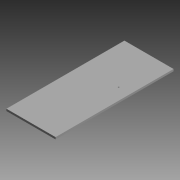
# Autodesk Inventor part: Wand rechts_CPY
Saved by Autodesk Inventor 2013 (Build 170138000, 138)
## iProperties
Created: 2012-10-20
Part Number: Wand rechts_CPY
Material: Allgemein
Document SubType Name: Modeling
Designer: fivef
Density: 1 g/cm^3
Author: fivef
Autodesk Inventor part; units mm, degrees
ref_plane "YZ Plane" through (0, 0, 0) normal (1, 0, 0) x (0, 1, 0)
ref_plane "XZ Plane" through (0, 0, 0) normal (0, 1, 0) x (-1, 0, 0)
ref_plane "XY Plane" through (0, 0, 0) normal (0, 0, 1) x (1, 0, 0)
sketch "Skizze1" plane through (0, 0, 0) normal (0, 0, 1) x (1, 0, 0)
  line L0 (0, 215.5102) -> (250, 215.5102)
  line L1 (250, 215.5102) -> (250, -384.4898)
  line L2 (250, -384.4898) -> (0, -384.4898)
  line L3 (0, -384.4898) -> (0, 215.5102)
  point P0 (0, 0)
  point P1 (190, -4.4898)
  dimension "d0" = 250
  dimension "d2" = 600
  dimension "d3" = 60
  dimension "d4" = 220
  constraints: 8 end point, 2 parallel, 1 horizontal, 1 perpendicular
  measures "d0" distance of L1.end L2.end
  measures "d2" distance of L0.end L1.end
  measures "d3" distance from line of L1 point (190, -4.49)
  measures "d4" distance from line of L0 point (190, -4.49)
extrude "Extrusion1" add sketch "Skizze1" along normal blind 10
hole "Bohrung1" at (190, -4.4898, 10) direction (0, 0, -1) diameter 6 end through all
